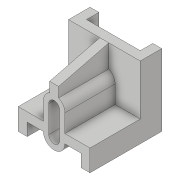
# Autodesk Inventor part: Part2
Saved by Autodesk Inventor 2017 (Build 210142000, 142)
## iProperties
Created: 2016-07-11
Part Number: Part2
Material: Generic
Document SubType Name: Modeling
Designer: anand
Density: 1 g/cm^3
Appearance: Default
Author: anand
Autodesk Inventor part; units mm, degrees
ref_plane "YZ Plane" through (0, 0, 0) normal (1, 0, 0) x (0, 1, 0)
ref_plane "XZ Plane" through (0, 0, 0) normal (0, 1, 0) x (-1, 0, 0)
ref_plane "XY Plane" through (0, 0, 0) normal (0, 0, 1) x (1, 0, 0)
sketch "Sketch1" plane through (0, 0, 0) normal (1, 0, 0) x (0, 1, 0)
  line L0 (0, 40.005) -> (0, 0)
  line L1 (0, 0) -> (40.005, 0)
  line L2 (40.005, 11.9888) -> (11.9888, 11.9888)
  line L3 (11.9888, 11.9888) -> (11.9888, 40.005)
  line L4 (40.005, 11.9888) -> (40.005, 0)
  line L5 (11.9888, 40.005) -> (0, 40.005)
  dimension "d0" = 40.005
  dimension "d1" = 40.005
  dimension "d2" = 11.9888
  constraints: 12 end point, 2 perpendicular, 2 vertical, 1 horizontal, 1 other
  measures "d0" distance of L0.end L1.end
  measures "d1" distance of L0.start L0.end
  measures "d2" distance of L3.end L0.start
extrude "Extrusion1" add sketch "Sketch1" along normal mid plane 40.005
shell "Shell1" thickness 5.0038 removed faces 4 at (6.6675, 40.005, 3.9963) at (6.6675, 13.335, 0) at (-6.6675, 3.9963, 40.005) at (6.6675, 0, 26.67)
sketch "Sketch2" plane through (-20.0025, 11.9888, 40.005) normal (0, 0, 1) x (1, 0, 0)
  line L0 (35.0012, -5.0038) -> (5.0038, -5.0038) projected
  line L1 (20.0152, -5.0038) -> (20.0152, 9.9822) construction
  line L2 (26.0096, -5.0038) -> (26.0096, 9.9822)
  line L3 (14.0208, 9.9822) -> (14.0208, -5.0038)
  arc A0 (14.0208, -5.0038) -> (26.0096, -5.0038) centre (20.0152, -5.0038) ccw
  arc A1 (26.0096, 9.9822) -> (14.0208, 9.9822) centre (20.0152, 9.9822) ccw
  line L4 (40.005, 0) -> (40.005, -11.9888) projected
  point P0 (20.0025, -11.9888)
  point P1 (20.0152, 2.4892)
  dimension "d6" = 5.9944
  dimension "d7" = 14.986
  dimension "d8" = 19.9898
  constraints: 8 end point, 4 point on circle, 4 tangent, 2 centre point, 1 midpoint, 1 parallel, 1 point on line, 1 vertical
  measures "d6" radius of A1
  measures "d7" distance of L2.start L2.end
  measures "d8" distance from line of L4 L1.start
extrude "Extrusion2" add sketch "Sketch2" against normal up to surface (33.02 mm away)
sketch "Sketch3" plane through (20.0025, 0, 40.005) normal (0, 0, 1) x (1, 0, 0)
  line L0 (-19.9898, 6.985) -> (-19.9898, 21.971) construction
  line L1 (-22.987, 6.985) -> (-22.987, 21.971)
  line L2 (-16.9926, 21.971) -> (-16.9926, 6.985)
  arc A0 (-22.987, 6.985) -> (-16.9926, 6.985) centre (-19.9898, 6.985) ccw
  arc A1 (-16.9926, 21.971) -> (-22.987, 21.971) centre (-19.9898, 21.971) ccw
  arc A2 (-13.9954, 21.971) -> (-25.9842, 21.971) centre (-19.9898, 21.971) ccw projected
  arc A3 (-25.9842, 6.985) -> (-13.9954, 6.985) centre (-19.9898, 6.985) ccw projected
  point P0 (-20.0025, 0)
  point P1 (-19.9898, 14.478)
  dimension "d12" = 2.9972
  constraints: 8 end point, 4 point on circle, 4 tangent, 2 centre point, 2 concentric, 1 midpoint, 1 parallel, 1 vertical
  measures "d12" radius of A0
extrude "Extrusion3" cut sketch "Sketch3" against normal through all
ref_plane "Work Plane1" through (0, 0, 0) normal (1, 0, 0) x (0, 0, -1)
sketch "Sketch4" plane through (0, 0, 0) normal (1, 0, 0) x (0, 0, -1)
  line L0 (-40.005, 27.9654) -> (-11.9888, 27.9654) projected
  line L1 (-11.9888, 27.9654) -> (-11.9888, 40.005) projected
  line L2 (-11.9888, 40.005) -> (-6.985, 40.005) projected
  line L3 (-6.985, 40.005) -> (-6.985, 24.9682) projected
  line L4 (-6.985, 24.9682) -> (-40.005, 24.9682) projected
  line L5 (-40.005, 24.9682) -> (-40.005, 27.9654) projected
  line L6 (-6.985, 0.9906) -> (-40.005, 0.9906) projected
  line L7 (-40.005, 0.9906) -> (-40.005, 3.9878) projected
  line L8 (-40.005, 3.9878) -> (-6.985, 3.9878) projected
  line L9 (-6.985, 3.9878) -> (-6.985, 0.9906) projected
  line L10 (-40.005, 27.9654) -> (-40.005, 32.9692)
  line L11 (-40.005, 32.9692) -> (-11.9888, 40.005)
  point P0 (0, 0)
  dimension "d15" = 5.0038
  constraints: 4 end point, 1 vertical
  measures "d15" distance of L0.start L10.end
extrude "Rib1" add sketch "Sketch4" along normal mid plane 5.0038 rib yes fills toward (-39.955, 30.4673) open curves L10 L11
body "Solid1"
